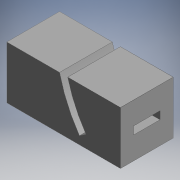
# Autodesk Inventor part: TestValve0
Saved by Autodesk Inventor 2018 (Build 220112000, 112)
## iProperties
Created: 2018-10-08
Part Number: TestValve0
Material: Generic
Document SubType Name: Modeling
Designer: Isaac Newcomb
Density: 1 g/cm^3
Appearance: Default
Author: Isaac Newcomb
Autodesk Inventor part; units mm, degrees
ref_plane "YZ Plane" through (0, 0, 0) normal (1, 0, 0) x (0, 1, 0)
ref_plane "XZ Plane" through (0, 0, 0) normal (0, 1, 0) x (-1, 0, 0)
ref_plane "XY Plane" through (0, 0, 0) normal (0, 0, 1) x (1, 0, 0)
sketch "Sketch1" plane through (0, 0, 0) normal (0, 0, 1) x (1, 0, 0)
  line L0 (0, 0) -> (21.5454, 0)
  line L1 (21.5454, 0) -> (21.5454, 10)
  line L2 (21.5454, 10) -> (11.5454, 10)
  line L3 (10, 10) -> (0, 10)
  line L4 (0, 10) -> (0, 0)
  arc A0 (10, 10) -> (13.7691, 1.5) centre (35, 16) ccw
  arc A1 (11.5454, 10) -> (15.0078, 2.346) centre (35, 16) ccw
  line L5 (15.0078, 2.346) -> (13.7691, 1.5)
  dimension "d0" = 10
  dimension "d2" = 10
  dimension "d4" = 10
  dimension "d11" = 1.5
  dimension "d12" = 1.5
  dimension "d13" = 35
  dimension "d14" = 16
  constraints: 12 end point, 4 point on circle, 3 perpendicular, 2 centre point, 2 point on line, 1 coincident, 1 horizontal, 1 line through centre
  measures "d0" distance of L3.end L0.start
  measures "d2" distance of L3.start L3.end
  measures "d4" distance of L1.end L2.end
  measures "d11" radial gap between concentric circles of A1 A0
  measures "d12" distance from line of L0 L5.end
  measures "d13" distance from line of L4 A0.centre
  measures "d14" distance from line of L0 A0.centre
extrude "Extrusion1" add sketch "Sketch1" along normal blind 10
sketch "Sketch2" plane through (21.5454, 0, 0) normal (1, 0, 0) x (0, 0, -1)
  line L0 (-10, 0) -> (0, 10) construction
  line L1 (-10, 10) -> (0, 0) construction
  line L2 (-7.5, 4.25) -> (-2.5, 4.25)
  line L3 (-2.5, 4.25) -> (-2.5, 5.75)
  line L4 (-2.5, 5.75) -> (-7.5, 5.75)
  line L5 (-7.5, 5.75) -> (-7.5, 4.25)
  line L6 (-7.5, 4.25) -> (-2.5, 5.75) construction
  line L7 (-2.5, 4.25) -> (-7.5, 5.75) construction
  point P0 (-5, 5)
  dimension "d7" = 5
  dimension "d8" = 1.5
  constraints: 16 end point, 3 midpoint, 2 parallel, 2 perpendicular, 1 horizontal
  measures "d7" distance of L4.end L3.end
  measures "d8" distance of L3.end L2.end
extrude "Extrusion2" cut sketch "Sketch2" against normal through all
body "Solid1"
